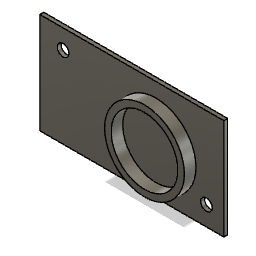
FM_door_assembly (Autodesk Fusion 360 archive; units mm, degrees)
design "boards setup_rfid_reader"
Autodesk Fusion 360 part; units mm, degrees
sketch "Sketch1" plane through (0, 0, 0) normal (0, 0, 1) x (1, 0, 0)
  line L0 (0, 0) -> (47.5, 0)
  line L1 (47.5, 0) -> (47.5, 26)
  line L2 (47.5, 26) -> (0, 26)
  line L3 (0, 26) -> (0, 0)
  circle A0 centre (6, 21) radius 1.5
  circle A1 centre (43, 5) radius 1.5
  dimension "d1" = 47.5
  dimension "d2" = 26
  dimension "d3" = 3
  dimension "d4" = 3
  dimension "d5" = 5
  dimension "d6" = 6
  dimension "d7" = 4.5
  dimension "d8" = 5
  dimension "d103" = 0
  dimension "d104" = 0
  dimension "d105" = 0
  dimension "d106" = 0
  dimension "d127" = 0
  dimension "d128" = 0
  dimension "d129" = 0
  dimension "d130" = 0
  constraint horizontal L0
  constraint vertical L1
  constraint horizontal L2
  constraint vertical L3
  constraint coincident L0.start L3.end
  measures "d1" distance of L0.start L0.end
  measures "d2" distance of L0.start L2.end
  measures "d3" diameter of A0
  measures "d4" diameter of A1
  measures "d5" distance of L2 A0.centre
  measures "d6" distance of L3 A0.centre
  measures "d7" distance of L1 A1.centre
  measures "d8" distance of L0 A1.centre
extrude "Extrude1" add sketch "Sketch1" along normal blind 1
sketch "Sketch2" plane through (0, 0, 1) normal (0, 0, 1) x (-1, 0, 0)
  circle A0 centre (-43, -5) radius 1.5
  circle A1 centre (-6, -21) radius 1.5
  line L0 (0, -26) -> (0, 0)
  line L1 (0, 0) -> (-47.5, 0)
  line L2 (-47.5, 0) -> (-47.5, -26)
  line L3 (-47.5, -26) -> (0, -26)
  circle A2 centre (-30, -12) radius 10.2956
  circle A3 centre (-30, -12) radius 8.6023
  dimension "d13" = 30
  constraint concentric A2 A3
  measures "d13" distance of L0 A2.centre
extrude "Extrude2" add sketch "Sketch2" along normal blind 3 contours A2
